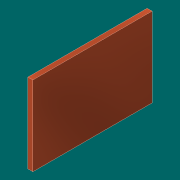
# Autodesk Inventor part: sides
Saved by Autodesk Inventor 2016 (Build 200138000, 138)
## iProperties
Created: 2015-10-13
Part Number: sides
Material: PC/ABS Plastic
Document SubType Name: Modeling
Designer: Sawaiz
Density: 0.357273 g/cm^3
Appearance: Copper - Polished
Author: Sawaiz
Autodesk Inventor part; units mm, degrees
ref_plane "YZ Plane" through (0, 0, 0) normal (1, 0, 0) x (0, 1, 0)
ref_plane "XZ Plane" through (0, 0, 0) normal (0, 1, 0) x (-1, 0, 0)
ref_plane "XY Plane" through (0, 0, 0) normal (0, 0, 1) x (1, 0, 0)
sketch "Sketch1" plane through (0, 0, 0) normal (0, 1, 0) x (-1, 0, 0)
  line L0 (-76.2, 50.8) -> (76.2, 50.8)
  line L1 (76.2, 50.8) -> (76.2, -50.8)
  line L2 (76.2, -50.8) -> (-76.2, -50.8)
  line L3 (-76.2, -50.8) -> (-76.2, 50.8)
  line L4 (-76.2, 50.8) -> (76.2, -50.8) construction
  line L5 (76.2, 50.8) -> (-76.2, -50.8) construction
  point P0 (0, 0)
  dimension "d0" = 152.4
  dimension "d1" = 101.6
  constraints: 12 end point, 2 midpoint, 2 parallel, 1 horizontal, 1 perpendicular
  measures "d0" distance of L1.end L2.end
  measures "d1" distance of L0.end L1.end
extrude "Extrusion1" add sketch "Sketch1" along normal blind 6.35
equation "\"d0\" = depth"
equation "\"d1\" = height"
equation "\"d2\" = acrylicThickness"
equation "\"acrylicThickness\" = 6.35"
equation "\"depth\" = 152.4"
equation "\"mirrorThickness\" = 3.175"
equation "\"height\" = 101.6"
equation "\"width\" = 101.6"
equation "\"mirrorAngle\" = 5deg"
equation "\"detectorWidth\" = 52"
equation "\"detectorHeight\" = 52"
equation "\"fresnelThickness\" = 0.1"
equation "\"focalLength\" = 76.2"
equation "\"ior\" = 1.49"
equation "\"centerThickness\" = 1.524"
equation "\"fresnelAngle\" = 90deg"
equation "\"fresnelEffectiveDiameter\" = 76.2"
equation "\"mirrorSuppourtWidth\" = 38.1"
equation "\"backGrooveBit\" = 4.8006"
equation "\"sensorHolderSensorWidth\" = 53.975"
equation "\"sensorHolderWidth\" = 88.9"
equation "\"sensorHolderSesnorHeight\" = 53.975"
equation "\"sensorHolderHeight\" = 88.9"
equation "\"sensorHolderSensorHeight\" = 53.975"
equation "\"sensorHolderORingGroove\" = 3.175"
equation "\"sensorHolderORing\" = 3.175"
equation "\"sensorHolderFlushORingID\" = 304.8"
equation "\"sensorHolderFlushORing\" = 3.175"
equation "\"frontBackORingID\" = 419.1"
equation "\"oRingWidth\" = 3.175"
equation "\"sensorHolderORingID\" = 203.2"
equation "\"topBottomHorizontalMirrorGroove\" = 12.7"
equation "\"backMirrorGroove\" = 6.35"
equation "\"mirrorGroove\" = 19.05"
equation "\"fresnelChamfer\" = 6.35"
equation "\"mirrorGrooveFillet\" = 6.35"
equation "\"mirrorGrooveDrill\" = 6.35"
equation "\"mirrorGrooveMill\" = 3.175"
equation "\"fresnelMirrorChamfer\" = 6.35"
equation "\"detectorOpeningHeight\" = 76.2"
equation "\"detectorOpeningWidth\" = 76.2"
body "Solid1"
